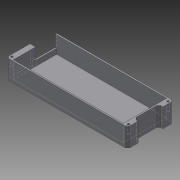
# Autodesk Inventor part: main body
Saved by Autodesk Inventor 2015 (Build 190159000, 159)
## iProperties
Created: 2019-05-11
Part Number: main body
Material: Generic
Document SubType Name: Modeling
Designer: Toby
Density: 1 g/cm^3
Appearance: Default
Author: Toby
Autodesk Inventor part; units mm, degrees
ref_plane "YZ Plane" through (0, 0, 0) normal (1, 0, 0) x (0, 1, 0)
ref_plane "XZ Plane" through (0, 0, 0) normal (0, 1, 0) x (-1, 0, 0)
ref_plane "XY Plane" through (0, 0, 0) normal (0, 0, 1) x (1, 0, 0)
sketch "Sketch1" plane through (0, 0, 0) normal (0, 0, 1) x (1, 0, 0)
  line L0 (-58.8402, 23.8593) -> (45.1598, 23.8593)
  line L1 (45.1598, 23.8593) -> (45.1598, -17.1407)
  line L2 (45.1598, -17.1407) -> (-58.8402, -17.1407)
  line L3 (-58.8402, -17.1407) -> (-58.8402, 23.8593)
  line L4 (-60.0402, 25.0593) -> (46.3598, 25.0593)
  line L5 (46.3598, 25.0593) -> (46.3598, -18.3407)
  line L6 (46.3598, -18.3407) -> (-60.0402, -18.3407)
  line L7 (-60.0402, -18.3407) -> (-60.0402, 25.0593)
  point P0 (0, 0)
  dimension "d0" = 104
  dimension "d1" = 41
  dimension "d2" = 1.2
  dimension "d3" = 1.2
  dimension "d4" = 1.2
  dimension "d5" = 1.2
  constraints: 16 end point, 4 parallel, 2 horizontal, 2 perpendicular
  measures "d0" distance of L0.start L0.end
  measures "d1" distance between parallel lines of L2 L0
  measures "d2" distance between parallel lines of L0 L4
  measures "d3" distance between parallel lines of L6 L2
  measures "d4" distance between parallel lines of L7 L3
  measures "d5" distance between parallel lines of L1 L5
extrude "Extrusion1" add sketch "Sketch1" along normal blind 16
sketch "Sketch2" plane through (0, 0, 0) normal (0, 0, -1) x (-1, 0, 0)
  line L0 (-46.3598, 25.0593) -> (60.0402, 25.0593)
  line L1 (60.0402, 25.0593) -> (60.0402, -18.3407)
  line L2 (60.0402, -18.3407) -> (-46.3598, -18.3407)
  line L3 (-46.3598, -18.3407) -> (-46.3598, 25.0593)
  point P0 (0, 0)
  constraints: 8 end point, 2 parallel, 1 horizontal, 1 perpendicular
extrude "Extrusion2" add sketch "Sketch2" along normal blind 2
sketch "Sketch3" plane through (0, 0, 16) normal (0, 0, 1) x (1, 0, 0)
  line L0 (-60.0402, 25.0593) -> (-60.0402, -18.3407) projected
  line L1 (-58.8402, 23.8593) -> (-60.0402, 23.8593)
  line L2 (-60.0402, 23.8593) -> (-60.0402, 3.8593)
  line L3 (-60.0402, 3.8593) -> (-58.8402, 3.8593)
  line L4 (-58.8402, 3.8593) -> (-58.8402, 23.8593)
  point P0 (0, 0)
  dimension "d10" = 20
  constraints: 8 end point, 2 parallel, 1 horizontal, 1 perpendicular, 1 point on line
  measures "d10" distance of L2.end L1.end
extrude "Extrusion3" cut sketch "Sketch3" against normal blind 11
sketch "Sketch4" plane through (0, 0, 16) normal (0, 0, 1) x (1, 0, 0)
  line L0 (-60.0402, -18.3407) -> (-64.0402, -18.3407)
  line L1 (-64.0402, -18.3407) -> (-64.0402, 3.8593)
  line L2 (-64.0402, 3.8593) -> (-60.0402, 3.8593)
  line L3 (-60.0402, 3.8593) -> (-60.0402, -18.3407)
  line L4 (-60.0402, 23.8593) -> (45.1598, 23.8593) projected
  line L5 (46.3598, 25.0593) -> (50.3598, 25.0593)
  line L6 (50.3598, 25.0593) -> (50.3598, 15.0593)
  line L7 (50.3598, 15.0593) -> (46.3598, 15.0593)
  line L8 (46.3598, 15.0593) -> (46.3598, 25.0593)
  line L9 (46.3598, -18.3407) -> (50.3598, -18.3407)
  line L10 (50.3598, -18.3407) -> (50.3598, -8.3407)
  line L11 (50.3598, -8.3407) -> (46.3598, -8.3407)
  line L12 (46.3598, -8.3407) -> (46.3598, -18.3407)
  point P0 (0, 0)
  dimension "d13" = 4
  dimension "d14" = 20
  dimension "d15" = 4
  dimension "d16" = 10
  dimension "d17" = 4
  dimension "d18" = 10
  constraints: 24 end point, 6 parallel, 3 horizontal, 3 perpendicular
  measures "d13" distance between parallel lines of L3 L1
  measures "d14" distance between parallel lines of L4 L2
  measures "d15" distance of L6.end L7.end
  measures "d16" distance of L5.end L6.end
  measures "d17" distance of L11.end L10.end
  measures "d18" distance of L10.end L9.end
extrude "Extrusion4" add sketch "Sketch4" against normal blind 18
chamfer "Chamfer1" distance 2 angle 45 1 edges at (-60.0402, 3.8593, 1.5)
chamfer "Chamfer2" distance 2 angle 45 2 edges at (46.3598, 15.0593, 7) (46.3598, -8.3407, 7)
sketch "Sketch5" plane through (0, 0, 16) normal (0, 0, 1) x (1, 0, 0)
  line L0 (-60.0402, 25.0593) -> (50.3598, 25.0593) projected
  line L1 (50.3598, 25.0593) -> (50.3598, 15.0593) projected
  line L2 (50.3598, -18.3407) -> (50.3598, -8.3407) projected
  line L3 (50.3598, -18.3407) -> (-64.0402, -18.3407) projected
  line L4 (-64.0402, -18.3407) -> (-64.0402, 3.8593) projected
  point P0 (0, 0)
  point P1 (-62.0402, -15.3407)
  point P2 (48.3598, -15.3407)
  point P3 (48.3598, 22.0593)
  dimension "d27" = 3
  dimension "d28" = 2
  dimension "d29" = 2
  dimension "d30" = 3
  dimension "d31" = 3
  dimension "d32" = 2
  dimension "d33" = 110.4
  dimension "d34" = 37.4
  measures "d27" distance from line of L0 point (48.36, 22.059)
  measures "d28" distance from line of L1 point (48.36, 22.059)
  measures "d29" distance from line of L2 point (48.36, -15.341)
  measures "d30" distance from line of L3 point (48.36, -15.341)
  measures "d31" distance from line of L3 point (-62.04, -15.341)
  measures "d32" distance from line of L4 point (-62.04, -15.341)
  measures "d33" distance of point (48.36, -15.341) point (-62.04, -15.341)
  measures "d34" distance of point (48.36, -15.341) point (48.36, 22.059)
hole "Hole1" at (-62.0402, -15.3407, 16) at (48.3598, -15.3407, 16) at (48.3598, 22.0593, 16) direction (0, 0, -1) diameter 2 depth 8 tip angle 118
chamfer "Chamfer3" distance 2 angle 45 3 edges at (50.3598, 25.0593, 7) (50.3598, -18.3407, 7) (-64.0402, -18.3407, 7)
body "Solid1"
